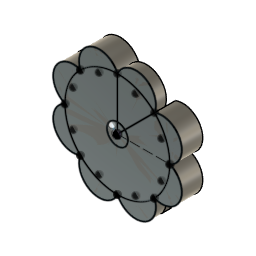
task2 v3 (Autodesk Fusion 360 design; units mm, degrees)
Autodesk Fusion 360 part; units mm, degrees
note: some values were not read from the file. Set by a fixed rule: which sketch regions a step uses.
sketch "Sketch1" plane through (0, 0, 0) normal (0, 1, 0) x (1, 0, 0)
  circle A0 centre (0, 0) radius 10
  circle A1 centre (0, 0) radius 50
  line L0 (0, 0) -> (50, 0) construction
  line L1 (-1.8153, 0) -> (-5, -5)
  line L2 (0, 0) -> (0, -50)
  line L3 (0, 0) -> (35.3553, -35.3553)
  arc A2 (0, -50) -> (35.3553, -35.3553) centre (17.4962, -42.2396) ccw
  arc A3 (35.3553, -35.3553) -> (50, 0) centre (42.2396, -17.4962) ccw
  arc A4 (50, 0) -> (35.3553, 35.3553) centre (42.2396, 17.4962) ccw
  arc A5 (35.3553, 35.3553) -> (0, 50) centre (17.4962, 42.2396) ccw
  arc A6 (0, 50) -> (-35.3553, 35.3553) centre (-17.4962, 42.2396) ccw
  arc A7 (-35.3553, 35.3553) -> (-50, 0) centre (-42.2396, 17.4962) ccw
  arc A8 (-50, 0) -> (-35.3553, -35.3553) centre (-42.2396, -17.4962) ccw
  arc A9 (-35.3553, -35.3553) -> (0, -50) centre (-17.4962, -42.2396) ccw
  dimension "d1" = 20
  dimension "d3" = 100
  dimension "d4" = 45
  dimension "d6" = 19.14
  dimension "d8" = 360
  constraint coincident A0.centre A1.centre
  constraint concentric A0 A1
  constraint coincident A1 L0.end
  constraint horizontal L0
  constraint coincident A1 L2.end
  constraint vertical L2
  constraint coincident A1 L3.end
  measures "d1" diameter of A0
  measures "d3" diameter of A1
  measures "d4" angle of L0 L3
  measures "d6" radius of A2
extrude "Extrude1" add sketch "Sketch1" along normal blind 20 makes body 1
extrude "Extrude2" cut sketch "Sketch1" against normal blind 10 from surface at 20 contours A0 L2 L3 | A0 A1 L2 L3 | A1 A2 picked at (2.9423, -5.9663) picked at (23.9603, -27.6522) bodies 1
pattern_circular "C-Pattern1" count 3 over 360 about axis through (0, 20, 0) along (0, -1, 0) of "Extrude2"
extrude "Extrude3" add sketch "Sketch1" along normal blind 10 separate body contours A0 L2 L3 | A0 L2 L3 makes body 2
